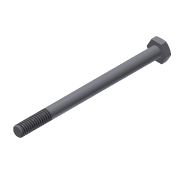
# Autodesk Inventor part: 250 hex bolt x4
Saved by Autodesk Inventor 2013 (Build 170138000, 138)
## iProperties
Created: 2011-07-11
Part Number: 250 hex bolt x4
Document SubType Name: Modeling
Designer: Dan Niemitalo
Density: 7.85 g/cm^3
Material: Steel
Mass: 28.4293 g
Surface Area: 23.605 cm^2
Volume: 3.62156 cm^3
Author: Dan Niemitalo
Autodesk Inventor part; units mm, degrees
ref_plane "YZ Plane" through (0, 0, 0) normal (1, 0, 0) x (0, 1, 0)
ref_plane "XZ Plane" through (0, 0, 0) normal (0, 1, 0) x (-1, 0, 0)
ref_plane "XY Plane" through (0, 0, 0) normal (0, 0, 1) x (1, 0, 0)
sketch "Sketch1" plane through (0, 0, 0) normal (0, 0, 1) x (1, 0, 0)
  circle A0 centre (0, 0) radius 3.175
  dimension "d0" = 6.35
  constraints: 1 centre point, 1 coincident
  measures "d0" diameter of A0
extrude "Extrusion1" add sketch "Sketch1" along normal blind 88.9
sketch "Sketch2" plane through (0, 0, 0) normal (0, 0, -1) x (-1, 0, 0)
  circle A0 centre (0, 0) radius 3.175 projected
  line L0 (-6.4158, 0) -> (-3.2079, 5.5563)
  line L1 (-3.2079, 5.5563) -> (3.2079, 5.5563)
  line L2 (3.2079, 5.5563) -> (6.4158, 0)
  line L3 (6.4158, 0) -> (3.2079, -5.5562)
  line L4 (3.2079, -5.5562) -> (-3.2079, -5.5563)
  line L5 (-3.2079, -5.5563) -> (-6.4158, 0)
  dimension "d3" = 11.1125
  constraints: 12 end point, 1 coincident, 1 horizontal, 13 other
  measures "d3" distance between parallel lines of L4 L1
extrude "Extrusion2" add sketch "Sketch2" along normal blind 3.9688 contours A0 | L0 L1 L2 L3 L4 L5
thread "Thread1" size "1/4-20 UNC" class "2A" standard "ANSI Unified Screw Threads" length 19.05
chamfer "Chamfer1" distance 0.508 angle 45 1 edges at (-3.175, 0, 88.9)
sketch "Sketch3" plane through (0, 0, 0) normal (0, 1, 0) x (-1, 0, 0)
  line L0 (-3.2079, -3.9688) -> (-6.4158, -3.9688) projected
  line L1 (-6.4158, 0) -> (-6.4158, -3.9688) projected
  line L2 (-3.2079, 0) -> (-6.4158, 0) projected
  line L3 (-3.2079, 0) -> (-3.2079, -3.9688) projected
  line L4 (3.2079, -3.9688) -> (-3.2079, -3.9688) projected
  line L5 (-3.2079, 0) -> (-3.2079, -3.9688) projected
  line L6 (3.2079, 0) -> (-3.2079, 0) projected
  line L7 (3.2079, 0) -> (3.2079, -3.9688) projected
  line L8 (0, -3.9688) -> (0, -7.4338)
  arc A0 (-6.4158, -3.0559) -> (-3.2079, -3.9688) centre (-3.2079, 2.1244) ccw
  line L9 (-3.2079, -3.9688) -> (-6.4158, -3.9688)
  line L10 (-6.4158, -3.9688) -> (-6.4158, -3.0559)
  point P0 (0, 0)
  constraints: 6 end point, 2 collinear, 2 point on circle, 2 tangent, 1 centre point, 1 midpoint, 1 parallel, 1 point on line
revolve "Revolution1" cut sketch "Sketch3" angle 360 about axis through (0, 0, -3.9688) along (0, 0, -1) contours L0 L1 A0
fillet "Fillet1" radius 0.254 18 edges at (3.2079, -5.5563, -1.528) (6.4158, 0, -1.528) (-3.2079, -5.5562, -1.528) (-6.4158, 0, -1.528) (-3.2079, 5.5563, -1.528) (3.2079, 5.5563, -1.528) (4.8119, 2.7781, 0) (0, 5.5563, 0) (-4.8119, 2.7781, 0) (-4.8119, -2.7781, 0) (0, -5.5562, 0) (4.8119, -2.7781, 0) (-4.8118, 2.7781, -3.498) (0, 5.5563, -3.498) (4.812, 2.778, -3.498) (4.812, -2.778, -3.498) (0, -5.5562, -3.498) (-4.8119, -2.7781, -3.498)
body "Solid1"
